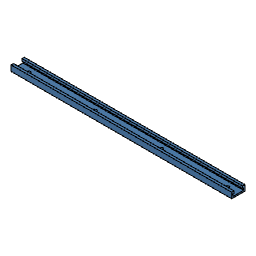
T-Track type 30 500mm (Autodesk Fusion 360 design; units mm, degrees)
Autodesk Fusion 360 part; units mm, degrees
sketch "T-track" plane through (0, 0, 0) normal (1, 0, 0) x (0, 1, 0)
  line L0 (-15, 0) -> (15, 0)
  line L1 (15, 0) -> (15, 12.8)
  line L2 (-15, 12.8) -> (-15, 0)
  line L3 (9.65, 12.8) -> (9.65, 7.8)
  line L4 (-9.65, 7.8) -> (-9.65, 12.8)
  line L5 (-12, 7.8) -> (-12, 3)
  line L6 (-12, 3) -> (12, 3)
  line L7 (12, 3) -> (12, 7.8)
  line L8 (15, 12.8) -> (9.65, 12.8)
  line L9 (-9.65, 12.8) -> (-15, 12.8)
  line L10 (12, 7.8) -> (9.65, 7.8)
  line L11 (-9.65, 7.8) -> (-12, 7.8)
  dimension "d1" = 30
  dimension "d2" = 12.8
  dimension "d3" = 19.3
  dimension "d4" = 5
  dimension "d5" = 9.65
  dimension "d6" = 24
  dimension "d7" = 4.8
  dimension "d8" = 12
  constraint horizontal L0
  constraint vertical L1
  constraint horizontal L8
  constraint vertical L2
  constraint vertical L3
  constraint vertical L4
  constraint coincident L4.end L8
  constraint horizontal L10
  constraint vertical L5
  constraint horizontal L6
  constraint vertical L7
  constraint collinear L8 L9
  constraint collinear L10 L11
  measures "d1" distance of L0.start L0.end
  measures "d2" distance of L0.start L2.start
  measures "d3" distance of L4.end L3.start
  measures "d4" distance of L4.end L4.start
  measures "d5" distance of origin L3
  measures "d6" distance of L7.end L5.start
  measures "d7" distance of L7.end L6.end
  measures "d8" distance of origin L7
  measures "d25" distance of L0.start
extrude "Extrude1" add sketch "T-track" along normal mid plane 500
sketch "Holes" plane through (0, 0, 3) normal (0, 0, 1) x (-1, 0, 0)
  line L0 (250, 12) -> (-250, 12)
  line L1 (-250, 12) -> (-250, -12)
  line L2 (-250, -12) -> (250, -12)
  line L3 (250, -12) -> (250, 12)
  line L4 (250, 0) -> (-250, 0) construction
  circle A0 centre (225, 0) radius 2
  circle A1 centre (-225, 0) radius 2
  circle A2 centre (-75, 0) radius 2
  circle A3 centre (75, 0) radius 2
  dimension "d12" = 4
  dimension "d13" = 4
  dimension "d14" = 25
  dimension "d22" = 4
  dimension "d23" = 4
  dimension "d24" = 150
  dimension "d25" = 150
  dimension "d26" = 150
  dimension "d27" = 25
  constraint midpoint L3 L4.start
  constraint midpoint L1 L4.end
  constraint coincident L4 A0.centre
  constraint coincident L4 A1.centre
  constraint coincident L4 A2.centre
  constraint coincident L4 A3.centre
  measures "d12" diameter of A0
  measures "d13" diameter of A1
  measures "d14" distance of L4.start A0.centre
  measures "d22" diameter of A2
  measures "d23" diameter of A3
  measures "d24" distance of A1.centre A2.centre
  measures "d25" distance of A2.centre A3.centre
  measures "d26" distance of A0.centre A3.centre
  measures "d27" distance of L1 A1.centre
extrude "Extrude2" cut sketch "Holes" against normal through all contours A0 | A1 | A2 | A3
chamfer "Chamfer2" distance 2 angle 45 4 edges at (226.8647, -0.7232, 3) (76.8647, -0.7232, 3) (-73.1353, -0.7232, 3) (-223.1353, -0.7232, 3)
equation "d5 = ( 19.3 / 2 ) * 1 mm"
equation "d8 = ( 24 / 2 ) * 1 mm"
equation "d12 = d13"
equation "d22 = d13"
equation "d23 = d13"
named bodies: "T-track"
